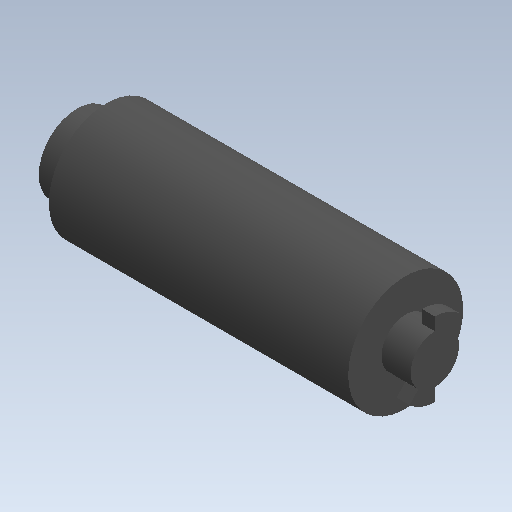
# Autodesk Inventor part: spool axle
Saved by Autodesk Inventor 2020.2 (Build 242310000, 310)
## iProperties
Created: 2020-02-09
Part Number: spool axle
Material: PLA
Document SubType Name: Modeling
Designer: mulve
Density: 1.3 g/cm^3
Appearance: Generic
Mass: 257.505 g
Surface Area: 218.205 cm^2
Volume: 198.081 cm^3
Author: mulve
Autodesk Inventor part; units mm, degrees
ref_plane "YZ Plane" through (0, 0, 0) normal (1, 0, 0) x (0, 1, 0)
ref_plane "XZ Plane" through (0, 0, 0) normal (0, 1, 0) x (-1, 0, 0)
ref_plane "XY Plane" through (0, 0, 0) normal (0, 0, 1) x (1, 0, 0)
sketch "Sketch1" plane through (0, 0, 0) normal (1, 0, 0) x (0, 1, 0)
  circle A0 centre (0, 0) radius 15
  dimension "d0" = 30
  constraints: 1 centre point, 1 coincident
  measures "d0" diameter of A0
extrude "Extrusion1" add sketch "Sketch1" along normal blind 140
sketch "Sketch2" plane through (140, 0, 0) normal (1, 0, 0) x (0, 0, -1)
  circle A0 centre (0, 0) radius 9.5
  circle A1 centre (0, 0) radius 15 projected
  line L0 (0, 15) -> (0, 9.5)
  line L1 (0, -9.5) -> (0, -15)
  line L2 (10.23, 10.9703) -> (6.479, 6.9479)
  line L3 (-10.23, -10.9703) -> (-6.479, -6.9479)
  dimension "d3" = 19
  dimension "d4" = 43
  dimension "d5" = 43
  constraints: 8 end point, 8 line through centre, 8 point on circle, 2 point on line, 1 centre point, 1 coincident, 1 vertical
  measures "d3" diameter of A0
  measures "d4" angle of L0 L2
  measures "d5" angle of L1 L3
extrude "Extrusion2" cut sketch "Sketch2" against normal blind 11.43 contours A0 L2 A1 L1 | A0 L3 A1 L0
sketch "Sketch3" plane through (128.57, 0, 0) normal (1, 0, 0) x (0, 0, -1)
  circle A0 centre (0, 0) radius 15
  circle A1 centre (0, 0) radius 9.5
  dimension "d22" = 19
  dimension "d23" = 30
  constraints: 2 centre point, 2 coincident
  measures "d22" diameter of A1
  measures "d23" diameter of A0
extrude "Extrusion3" cut sketch "Sketch3" along normal blind 6.35
sketch "Sketch6" plane through (0, 0, 0) normal (-1, 0, 0) x (0, 0, 1)
  circle A0 centre (0, 0) radius 22.5
  dimension "d16" = 45
  constraints: 1 centre point, 1 coincident
  measures "d16" diameter of A0
extrude "Extrusion6" add sketch "Sketch6" against normal up to surface (128.57 mm away)
sketch "Sketch7" plane through (0, 0, 0) normal (-1, 0, 0) x (0, 0, 1)
  circle A0 centre (0, 0) radius 15
  circle A1 centre (0, 0) radius 22.5
  dimension "d19" = 30
  constraints: 2 centre point, 2 coincident
  measures "d19" diameter of A0
extrude "Extrusion7" cut sketch "Sketch7" against normal blind 11.43
sketch "Sketch8" plane through (140, 0, 0) normal (1, 0, 0) x (0, 0, -1)
  arc A0 (10.23, 10.9703) -> (0, 15) centre (0, 0) ccw projected
  circle A1 centre (0, 0) radius 15
  circle A2 centre (0, 0) radius 14.5
  point P0 (0, 15)
  dimension "d24" = 0.5
  constraints: 2 coincident, 1 centre point, 3 other
extrude "Extrusion8" cut sketch "Sketch8" against normal up to surface (5.08 mm away)
body "Solid1"
